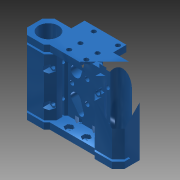
# Autodesk Inventor part: ChimeraXCarriage5
Saved by Autodesk Inventor 2015 SP1 (Build 190203100, 203)
## iProperties
Created: 2015-03-08
Part Number: ChimeraXCarriage5
Material: ABS Plastic
Document SubType Name: Modeling
Designer: Jack
Density: 1.06 g/cm^3
Appearance: Cyan
Author: Jack
Autodesk Inventor part; units mm, degrees
ref_plane "YZ Plane" through (0, 0, 0) normal (1, 0, 0) x (0, 1, 0)
ref_plane "XZ Plane" through (0, 0, 0) normal (0, 1, 0) x (-1, 0, 0)
ref_plane "XY Plane" through (0, 0, 0) normal (0, 0, 1) x (1, 0, 0)
sketch "Sketch2" plane through (0, 0, 0) normal (0, 0, 1) x (1, 0, 0)
  arc A0 (7.6035, 1.5) -> (7.6035, -1.5) centre (0, 0) ccw
  arc A1 (47.3965, -1.5) -> (47.3965, 1.5) centre (55, 0) ccw
  line L0 (-11, -11) -> (-11, 11)
  line L1 (66, 11) -> (66, -11)
  line L2 (66, -11) -> (42.5, -11)
  line L3 (42.5, -11) -> (42.5, -1.5)
  line L4 (42.5, -1.5) -> (47.3965, -1.5)
  line L5 (-11, -11) -> (12.5, -11)
  line L6 (12.5, -11) -> (12.5, -1.5)
  line L7 (7.6035, -1.5) -> (12.5, -1.5)
  line L8 (-11, 11) -> (66, 11)
  line L9 (7.6035, 1.5) -> (12.5, 1.5)
  line L10 (12.5, 1.5) -> (12.5, 3)
  line L11 (12.5, 3) -> (42.5, 3)
  line L12 (42.5, 3) -> (42.5, 1.5)
  line L13 (42.5, 1.5) -> (47.3965, 1.5)
  dimension "d11" = 15.5
  dimension "d12" = 55
  dimension "d13" = 11
  dimension "d15" = 11
  dimension "d17" = 1.5
  dimension "d18" = 12.5
  dimension "d19" = 12.5
  dimension "d20" = 11
  dimension "d29" = 1.5
  dimension "d30" = 8
  constraints: 28 end point, 6 perpendicular, 5 point on circle, 4 horizontal, 3 point on line, 2 centre point, 2 collinear, 2 horizontal alignment, 2 vertical, 1 coincident, 1 equal radius, 1 parallel, 1 vertical alignment
  measures "d11" diameter of A0
  measures "d12" distance of A1.centre point (0, 0)
  measures "d13" distance from line of L5 point (0, 0)
  measures "d15" distance from line of point (0, 0) L0
  measures "d17" distance from line of point (0, 0) L7
  measures "d18" distance from line of point (0, 0) L6
  measures "d19" distance from line of A1.centre L3
  measures "d20" distance from line of point (0, 0) L8
  measures "d29" distance from line of point (0, 0) L9
  measures "d30" distance between parallel lines of L8 L11
extrude "Extrusion1" add sketch "Sketch2" along normal blind 48
chamfer "Chamfer1" distance 5 angle 45 2 edges at (12.5, -11, 24) (42.5, -11, 24)
chamfer "Chamfer2" distance 5 angle 45 4 edges at (-11, -11, 24) (-11, 11, 24) (66, 11, 24) (66, -11, 24)
sketch "Sketch6" plane through (0, 0, 0) normal (0, 0, -1) x (-1, 0, 0)
  line L0 (-61, -11) -> (-66, -6) projected
  line L1 (-61, -11) -> (-47.5, -11) projected
  line L2 (-42.5, -6) -> (-42.5, -1.5) projected
  line L3 (-42.5, -1.5) -> (-47.3965, -1.5) projected
  arc A0 (-47.3965, 1.5) -> (-47.3965, -1.5) centre (-55, 0) ccw projected
  line L4 (-47.3965, 1.5) -> (-42.5, 1.5) projected
  line L5 (-42.5, 1.5) -> (-42.5, 3) projected
  line L6 (-42.5, 3) -> (-12.5, 3) projected
  line L7 (-12.5, 3) -> (-12.5, 1.5) projected
  line L8 (-12.5, 1.5) -> (-7.6035, 1.5) projected
  arc A1 (-7.6035, -1.5) -> (-7.6035, 1.5) centre (0, 0) ccw projected
  line L9 (-7.6035, -1.5) -> (-12.5, -1.5) projected
  line L10 (-12.5, -1.5) -> (-12.5, -6) projected
  line L11 (-7.5, -11) -> (6, -11) projected
  line L12 (11, -6) -> (6, -11) projected
  line L13 (11, -6) -> (11, 6) projected
  line L14 (6, 11) -> (11, 6) projected
  line L15 (6, 11) -> (-61, 11) projected
  line L16 (-66, 6) -> (-61, 11) projected
  line L17 (-66, 6) -> (-66, -6) projected
  line L18 (-47.5, -11) -> (-42.5, -6) projected
  line L19 (-45.2, -8.7) -> (-9.8, -8.7)
  line L20 (-12.5, -6) -> (-7.5, -11) projected
  arc A2 (-47.3965, -1.5) -> (-47.3965, 1.5) centre (-55, 0) ccw
  arc A3 (-7.6035, 1.5) -> (-7.6035, -1.5) centre (0, 0) ccw
  dimension "d37" = 8.7
  constraints: 4 point on circle, 2 centre point, 2 coincident, 2 end point, 2 point on line, 1 horizontal
  measures "d37" distance from line of A0.centre L19
extrude "Extrusion4" add sketch "Sketch6" along normal blind 5 contours L0 L17 L16 L15 L14 L13 L12 L11 L20 L10 L9 A1 L8 L7 L6 L5 L4 A0 L3 L2 L18 L1 | L18 L2 L3 A2 L4 L5 L6 L7 L8 A3 L9 L10 L20 L19
sketch "Sketch7" plane through (0, 0, 48) normal (0, 0, 1) x (1, 0, 0)
  line L0 (66, -6) -> (61, -11) projected
  line L1 (66, -6) -> (66, 6) projected
  line L2 (61, 11) -> (66, 6) projected
  line L3 (61, 11) -> (-6, 11) projected
  line L4 (-11, 6) -> (-6, 11) projected
  line L5 (-11, 6) -> (-11, -6) projected
  line L6 (-6, -11) -> (-11, -6) projected
  line L7 (-6, -11) -> (7.5, -11) projected
  line L8 (12.5, -6) -> (7.5, -11) projected
  line L9 (12.5, -6) -> (12.5, -1.5) projected
  line L10 (12.5, -1.5) -> (7.6035, -1.5) projected
  arc A0 (7.6035, 1.5) -> (7.6035, -1.5) centre (0, 0) ccw projected
  line L11 (7.6035, 1.5) -> (12.5, 1.5) projected
  line L12 (12.5, 1.5) -> (12.5, 3) projected
  line L13 (12.5, 3) -> (42.5, 3) projected
  line L14 (42.5, 3) -> (42.5, 1.5) projected
  line L15 (42.5, 1.5) -> (47.3965, 1.5) projected
  arc A1 (47.3965, -1.5) -> (47.3965, 1.5) centre (55, 0) ccw projected
  line L16 (47.3965, -1.5) -> (42.5, -1.5) projected
  line L17 (42.5, -1.5) -> (42.5, -6) projected
  line L18 (47.5, -11) -> (42.5, -6) projected
  line L19 (47.5, -11) -> (61, -11) projected
  line L20 (42.5, -6) -> (45.2, -8.7) projected
  line L21 (42.5, -6) -> (42.5, -1.5) projected
  line L22 (42.5, -1.5) -> (47.3965, -1.5) projected
  arc A2 (47.3965, 1.5) -> (47.3965, -1.5) centre (55, 0) ccw projected
  line L23 (47.3965, 1.5) -> (42.5, 1.5) projected
  line L24 (42.5, 1.5) -> (42.5, 3) projected
  line L25 (42.5, 3) -> (12.5, 3) projected
  line L26 (12.5, 3) -> (12.5, 1.5) projected
  line L27 (12.5, 1.5) -> (7.6035, 1.5) projected
  arc A3 (7.6035, -1.5) -> (7.6035, 1.5) centre (0, 0) ccw projected
  line L28 (7.6035, -1.5) -> (12.5, -1.5) projected
  line L29 (12.5, -1.5) -> (12.5, -6) projected
  line L30 (9.8, -8.7) -> (12.5, -6) projected
  line L31 (45.2, -8.7) -> (9.8, -8.7) projected
extrude "Extrusion5" add sketch "Sketch7" along normal blind 5 contours L0 L19 L18 L17 L16 A1 L15 L14 L13 L12 L11 A0 L10 L9 L8 L7 L6 L5 L4 L3 L2 L1 | L31 L8 L9 L10 A3 L11 L12 L13 L14 L15 A2 L16 L17 L18
sketch "Sketch8" plane through (-11, -6, -5) normal (-1, 0, 0) x (0, 0, 1)
  line L0 (5, 4.5) -> (53, 4.5) projected
  line L1 (0, -5) -> (58, -5) projected
  line L2 (53, 4.5) -> (53, -5)
  line L3 (58, -5) -> (0, -5) projected
  line L4 (51.5, 4.5) -> (51.5, -5)
  point P0 (5, 6)
  dimension "d42" = 1.5
  constraints: 4 end point, 3 point on line, 2 perpendicular
  measures "d42" distance between parallel lines of L2 L4
extrude "Extrusion6" cut sketch "Sketch8" against normal up to surface (23.5 mm away)
sketch "Sketch9" plane through (-11, -6, -5) normal (-1, 0, 0) x (0, 0, 1)
  line L0 (0, -5) -> (51.5, -5) projected
  line L1 (5, 4.5) -> (51.5, 4.5) projected
  line L2 (6.5, 4.5) -> (6.5, -5)
  line L3 (51.5, -5) -> (0, -5) projected
  line L4 (5, 4.5) -> (5, -5)
  point P0 (5, 6)
  dimension "d45" = 1.5
  constraints: 4 end point, 3 point on line, 2 perpendicular
  measures "d45" distance between parallel lines of L4 L2
extrude "Extrusion7" cut sketch "Sketch9" against normal up to surface (23.5 mm away)
sketch "Sketch10" plane through (66, -6, -5) normal (1, 0, 0) x (0, 0, -1)
  line L0 (-5, 4.5) -> (-53, 4.5) projected
  line L1 (-58, -5) -> (0, -5) projected
  line L2 (-53, 4.5) -> (-53, -5)
  line L3 (-53, -5) -> (-53, -2.7) projected
  line L4 (-5, 4.5) -> (-5, -5)
  line L5 (0, -5) -> (-58, -5) projected
  line L6 (-6.5, 4.5) -> (-51.5, 4.5) projected
  line L7 (-6.5, 4.5) -> (-6.5, -5)
  line L8 (-51.5, -5) -> (-6.5, -5) projected
  line L9 (-51.5, 4.5) -> (-51.5, -5)
  point P0 (-5, 6)
  dimension "d48" = 1.5
  dimension "d49" = 1.5
  constraints: 8 end point, 5 point on line, 2 perpendicular, 1 collinear, 1 vertical
  measures "d48" distance between parallel lines of L2 L9
  measures "d49" distance between parallel lines of L4 L7
extrude "Extrusion8" cut sketch "Sketch10" against normal up to surface (23.5 mm away) contours L4 L1 L7 L0 | L9 L1 L2 L0
chamfer "Chamfer3" distance 1.5 angle 45 2 edges at (12.5, 1.5, 24) (42.5, 1.5, 24)
sketch "Sketch11" plane through (-6, -11, 46.5) normal (0, -1, 0) x (1, 0, 0)
  line L0 (18.5, -45) -> (18.5, 0) projected
  line L1 (48.5, 0) -> (48.5, -45) projected
  line L2 (53.5, -45) -> (53.5, 0) projected
  circle A0 centre (15.5, -10) radius 1.75
  circle A1 centre (15.5, -35) radius 1.75
  circle A2 centre (51, -35) radius 1.75
  circle A3 centre (51, -10) radius 1.75
  line L3 (53.5, 0) -> (48.5, 0) projected
  line L4 (48.5, -45) -> (53.5, -45) projected
  point P0 (6, -46.5)
  dimension "d55" = 3.5
  dimension "d56" = 3
  dimension "d57" = 2.5
  dimension "d58" = 10
  dimension "d59" = 10
  constraints: 4 centre point, 3 equal radius, 2 horizontal alignment, 2 vertical alignment
  measures "d55" diameter of A0
  measures "d56" distance from line of L0 A1.centre
  measures "d57" distance from line of L1 A3.centre
  measures "d58" distance from line of L3 A3.centre
  measures "d59" distance from line of L4 A2.centre
extrude "Extrusion9" cut sketch "Sketch11" against normal up to surface (22 mm away) contours A0 | A1 | A2 | A3
sketch "Sketch12" plane through (-6, 11, -5) normal (0, 1, 0) x (1, 0, 0)
  circle A0 centre (51, -16.5) radius 1.75 projected
  circle A1 centre (51, -41.5) radius 1.75 projected
  circle A2 centre (15.5, -16.5) radius 1.75 projected
  circle A3 centre (15.5, -41.5) radius 1.75 projected
  circle A4 centre (15.5, -16.5) radius 3
  circle A5 centre (15.5, -41.5) radius 3
  circle A6 centre (51, -16.5) radius 3
  circle A7 centre (51, -41.5) radius 3
  point P0 (6, -5)
  dimension "d62" = 6
  constraints: 4 centre point, 4 coincident, 3 equal radius
  measures "d62" diameter of A4
extrude "Extrusion10" cut sketch "Sketch12" against normal blind 3.5
sketch "Sketch13" plane through (-6, -11, 46.5) normal (0, -1, 0) x (1, 0, 0)
  circle A0 centre (15.5, -10) radius 1.75 projected
  circle A1 centre (15.5, -35) radius 1.75 projected
  circle A2 centre (51, -10) radius 1.75 projected
  circle A3 centre (51, -35) radius 1.75 projected
  line L0 (15.5, -6.8246) -> (18.25, -8.4123)
  line L1 (18.25, -8.4123) -> (18.25, -11.5877)
  line L2 (18.25, -11.5877) -> (15.5, -13.1754)
  line L3 (15.5, -13.1754) -> (12.75, -11.5877)
  line L4 (12.75, -11.5877) -> (12.75, -8.4123)
  line L5 (12.75, -8.4123) -> (15.5, -6.8246)
  line L6 (15.5, -31.8246) -> (18.25, -33.4123)
  line L7 (18.25, -33.4123) -> (18.25, -36.5877)
  line L8 (18.25, -36.5877) -> (15.5, -38.1754)
  line L9 (15.5, -38.1754) -> (12.75, -36.5877)
  line L10 (12.75, -36.5877) -> (12.75, -33.4123)
  line L11 (12.75, -33.4123) -> (15.5, -31.8246)
  line L12 (51, -31.8246) -> (53.75, -33.4123)
  line L13 (53.75, -33.4123) -> (53.75, -36.5877)
  line L14 (53.75, -36.5877) -> (51, -38.1754)
  line L15 (51, -38.1754) -> (48.25, -36.5877)
  line L16 (48.25, -36.5877) -> (48.25, -33.4123)
  line L17 (48.25, -33.4123) -> (51, -31.8246)
  line L18 (51, -6.8246) -> (53.75, -8.4123)
  line L19 (53.75, -8.4123) -> (53.75, -11.5877)
  line L20 (53.75, -11.5877) -> (51, -13.1754)
  line L21 (51, -13.1754) -> (48.25, -11.5877)
  line L22 (48.25, -11.5877) -> (48.25, -8.4123)
  line L23 (48.25, -8.4123) -> (51, -6.8246)
  point P0 (6, -46.5)
  dimension "d65" = 5.5
  constraints: 48 end point, 4 coincident, 4 vertical, 3 equal length, 52 other
  measures "d65" distance between parallel lines of L4 L1
extrude "Extrusion11" cut sketch "Sketch13" against normal blind 5 contours A0 | A1 | A2 | A3 | L0 L1 L2 L3 L4 L5 | L6 L7 L8 L9 L10 L11 | L12 L13 L14 L15 L16 L17 | L18 L19 L20 L21 L22 L23
sketch "Sketch14" plane through (47.5, -11, 1.5) normal (0, -1, 0) x (1, 0, 0)
  line L0 (-5, 33.2679) -> (-5, 11.7321) projected
  line L1 (-5, 31.5) -> (-2.5, 31.5)
  line L2 (-2.5, 31.5) -> (-2.5, 13.5)
  line L3 (-2.5, 13.5) -> (-5, 13.5)
  line L4 (-5, 0) -> (0, 0) projected
  line L5 (0, 45) -> (-5, 45) projected
  point P0 (-47.5, -1.5)
  dimension "d68" = 2.5
  dimension "d69" = 13.5
  dimension "d70" = 13.5
  constraints: 6 end point, 2 perpendicular, 2 point on line, 1 horizontal
  measures "d68" distance of L2.end L3.end
  measures "d69" distance between parallel lines of L4 L3
  measures "d70" distance between parallel lines of L5 L1
extrude "Extrusion12" cut sketch "Sketch14" against normal up to surface (9.5 mm away)
chamfer "Chamfer4" distance 1 angle 45 2 edges at (45, -5, 15) (45, -5, 33)
sketch "Sketch15" plane through (12.5, 3, 0) normal (0, -1, 0) x (1, 0, 0)
  line L0 (0, 48) -> (30, 48) projected
  line L1 (0, 0) -> (0, 48) projected
  circle A0 centre (15, 32.5) radius 1.75
  circle A1 centre (15, 15.5) radius 1.75
  circle A2 centre (3, 24) radius 1.75
  point P0 (-12.5, 0)
  dimension "d76" = 3.5
  dimension "d77" = 15
  dimension "d78" = 17
  dimension "d79" = 15.5
  dimension "d116" = 12
  dimension "d117" = 8.5
  constraints: 3 centre point, 2 equal radius, 1 vertical alignment
  measures "d76" diameter of A0
  measures "d77" distance from line of L1 A0.centre
  measures "d78" distance of A1.centre A0.centre
  measures "d79" distance from line of L0 A0.centre
  measures "d116" horizontal distance of A0.centre A2.centre
  measures "d117" vertical distance of A1.centre A2.centre
extrude "Extrusion13" cut sketch "Sketch15" against normal up to next
sketch "Sketch16" plane through (-6, 11, -5) normal (0, 1, 0) x (1, 0, 0)
  circle A0 centre (33.5, -37.5) radius 1.75 projected
  arc A1 (28.327, -36.8365) -> (21.273, -40.3635) centre (24.5, -38) ccw
  arc A2 (21.273, -17.6365) -> (28.327, -21.1635) centre (24.5, -20) ccw
  arc A3 (26.4831, -47.4772) -> (30.8919, -45.2728) centre (28.5, -46) ccw
  arc A4 (30.8919, -12.7272) -> (26.4831, -10.5228) centre (28.5, -12) ccw
  line L0 (30.8919, -45.2728) -> (28.327, -36.8365)
  line L1 (26.4831, -47.4772) -> (21.273, -40.3635)
  line L2 (30.8919, -12.7272) -> (28.327, -21.1635)
  line L3 (26.4831, -10.5228) -> (21.273, -17.6365)
  circle A5 centre (21.5, -29) radius 1.75 projected
  point P0 (6, -5)
  dimension "d82" = 8
  dimension "d86" = 5
  dimension "d87" = 8
  dimension "d88" = 4
  dimension "d89" = 8
  dimension "d119" = 18
  dimension "d120" = 9
  dimension "d121" = 9
  constraints: 8 end point, 8 point on circle, 8 tangent, 4 centre point, 2 equal radius, 2 vertical alignment
  measures "d82" diameter of A1
  measures "d86" diameter of A3
  measures "d87" vertical distance of A2.centre A4.centre
  measures "d88" horizontal distance of A2.centre A4.centre
  measures "d89" vertical distance of A1.centre A3.centre
  measures "d119" distance of A2.centre A1.centre
  measures "d120" vertical distance of A5.centre A1.centre
  measures "d121" horizontal distance of A0.centre A1.centre
extrude "Extrusion14" cut sketch "Sketch16" against normal up to next contours L0 A3 L1 A1 | L3 A4 L2 A2
sketch "Sketch17" plane through (-6, 11, -5) normal (0, 1, 0) x (1, 0, 0)
  circle A0 centre (33.5, -37.5) radius 1.75 projected
  circle A1 centre (33.5, -20.5) radius 1.75 projected
  circle A2 centre (33.5, -37.5) radius 3
  circle A3 centre (33.5, -20.5) radius 3
  circle A4 centre (21.5, -29) radius 1.75 projected
  circle A5 centre (21.5, -29) radius 3
  point P0 (6, -5)
  dimension "d90" = 6
  constraints: 3 centre point, 3 coincident, 2 equal radius
  measures "d90" diameter of A2
extrude "Extrusion15" cut sketch "Sketch17" against normal blind 3.5
sketch "Sketch18" plane through (0, 0, 53) normal (0, 0, 1) x (1, 0, 0)
  circle A0 centre (0, 0) radius 7.75 projected
  circle A1 centre (20.75, -4.45) radius 1.75
  circle A2 centre (34.25, -4.45) radius 1.75
  circle A3 centre (34.25, 4.45) radius 1.75
  circle A4 centre (20.75, 4.45) radius 1.75
  dimension "d93" = 3.5
  dimension "d94" = 13.5
  dimension "d95" = 8.9
  dimension "d96" = 20.75
  dimension "d97" = 4.45
  constraints: 4 centre point, 3 equal radius, 2 horizontal alignment, 2 vertical alignment
  measures "d93" diameter of A1
  measures "d94" distance of A3.centre A4.centre
  measures "d95" distance of A4.centre A1.centre
  measures "d96" horizontal distance of A0.centre A1.centre
  measures "d97" vertical distance of A0.centre A1.centre
extrude "Extrusion16" cut sketch "Sketch18" against normal up to surface (5 mm away) contours A1 | A2 | A3 | A4
sketch "Sketch19" plane through (0, 0, -5) normal (0, 0, -1) x (-1, 0, 0)
  circle A0 centre (-20.75, -4.45) radius 1.75 projected
  circle A1 centre (-20.75, 4.45) radius 1.75 projected
  circle A2 centre (-34.25, 4.45) radius 1.75 projected
  circle A3 centre (-34.25, -4.45) radius 1.75 projected
extrude "Extrusion17" cut sketch "Sketch19" against normal up to surface (5 mm away)
sketch "Sketch20" plane through (20.75, 4.45, 0) normal (0, 0, -1) x (-1, 0, 0)
  line L0 (-0.9798, -1.45) -> (0.9798, -1.45) projected
  arc A0 (0.9798, -1.45) -> (-0.9798, -1.45) centre (0, 0) ccw projected
  line L1 (-14.4798, -1.45) -> (-12.5202, -1.45) projected
  arc A1 (-12.5202, -1.45) -> (-14.4798, -1.45) centre (-13.5, 0) ccw projected
  line L2 (-10.75, -1.5877) -> (-13.5, -3.1754)
  line L3 (-13.5, -3.1754) -> (-16.25, -1.5877)
  line L4 (-16.25, -1.5877) -> (-16.25, 1.5877)
  line L5 (-16.25, 1.5877) -> (-13.5, 3.1754)
  line L6 (-13.5, 3.1754) -> (-10.75, 1.5877)
  line L7 (-10.75, 1.5877) -> (-10.75, -1.5877)
  line L8 (-2.75, -1.5877) -> (-2.75, 1.5877)
  line L9 (-2.75, 1.5877) -> (0, 3.1754)
  line L10 (0, 3.1754) -> (2.75, 1.5877)
  line L11 (2.75, 1.5877) -> (2.75, -1.5877)
  line L12 (2.75, -1.5877) -> (0, -3.1754)
  line L13 (0, -3.1754) -> (-2.75, -1.5877)
  point P0 (20.75, -4.45)
  point P1 (-13.5, 0)
  dimension "d102" = 5.5
  constraints: 24 end point, 2 coincident, 2 vertical, 1 parallel, 26 other
  measures "d102" distance between parallel lines of L3 L6
extrude "Extrusion18" cut sketch "Sketch20" along normal blind 3 and the other way blind 3 contours A0 L0 | A1 L1 | L2 L3 L4 L5 L6 L7 | L8 L9 L10 L11 L12 L13
sketch "Sketch21" plane through (34.25, 4.45, 48) normal (0, 0, 1) x (1, 0, 0)
  line L0 (-14.4798, -1.45) -> (-12.5202, -1.45) projected
  arc A0 (-12.5202, -1.45) -> (-14.4798, -1.45) centre (-13.5, 0) ccw projected
  circle A1 centre (-13.5, 0) radius 1.75 projected
  line L1 (-10.75, 1.5877) -> (-10.75, -1.5877) projected
  line L2 (-13.5, 3.1754) -> (-10.75, 1.5877) projected
  line L3 (-16.25, 1.5877) -> (-13.5, 3.1754) projected
  line L4 (-16.25, -1.5877) -> (-16.25, 1.5877) projected
  line L5 (-13.5, -3.1754) -> (-16.25, -1.5877) projected
  line L6 (-10.75, -1.5877) -> (-13.5, -3.1754) projected
  circle A2 centre (0, 0) radius 1.75 projected
  line L7 (0, -3.1754) -> (-2.75, -1.5877) projected
  line L8 (2.75, -1.5877) -> (0, -3.1754) projected
  line L9 (2.75, 1.5877) -> (2.75, -1.5877) projected
  line L10 (0, 3.1754) -> (2.75, 1.5877) projected
  line L11 (-2.75, 1.5877) -> (0, 3.1754) projected
  line L12 (-2.75, -1.5877) -> (-2.75, 1.5877) projected
  point P0 (-34.25, -4.45)
extrude "Extrusion19" cut sketch "Sketch21" along normal blind 3 and the other way blind 3 contours A0 L0 | L1 L6 L5 L4 L3 L2 | A2 | L7 L12 L11 L10 L9 L8
sketch "Sketch22" plane through (0, 0, 48) normal (0, 0, -1) x (-1, 0, 0)
  circle A0 centre (-20.75, -4.45) radius 1.75 projected
  circle A1 centre (-34.25, -4.45) radius 1.75 projected
  line L0 (-18, 2.8623) -> (-20.75, 1.2746) projected
  line L1 (-20.75, -7.6254) -> (-23.5, -6.0377)
  line L2 (-23.5, -6.0377) -> (-23.5, -2.8623)
  line L3 (-23.5, -2.8623) -> (-20.75, -1.2746)
  line L4 (-20.75, -1.2746) -> (-18, -2.8623)
  line L5 (-18, -2.8623) -> (-18, -6.0377)
  line L6 (-18, -6.0377) -> (-20.75, -7.6254)
  line L7 (-34.25, -7.6254) -> (-37, -6.0377)
  line L8 (-37, -6.0377) -> (-37, -2.8623)
  line L9 (-37, -2.8623) -> (-34.25, -1.2746)
  line L10 (-34.25, -1.2746) -> (-31.5, -2.8623)
  line L11 (-31.5, -2.8623) -> (-31.5, -6.0377)
  line L12 (-31.5, -6.0377) -> (-34.25, -7.6254)
  constraints: 24 end point, 2 coincident, 2 equal length, 2 vertical, 26 other
extrude "Extrusion20" cut sketch "Sketch22" against normal blind 3
sketch "Sketch23" plane through (0, 0, 0) normal (0, 0, 1) x (1, 0, 0)
  circle A0 centre (20.75, -4.45) radius 1.75 projected
  circle A1 centre (34.25, -4.45) radius 1.75 projected
  circle A2 centre (20.75, -4.45) radius 1.75 projected
  line L0 (20.75, -7.6254) -> (23.5, -6.0377) projected
  line L1 (18, -6.0377) -> (20.75, -7.6254) projected
  line L2 (18, -2.8623) -> (18, -6.0377) projected
  line L3 (20.75, -1.2746) -> (18, -2.8623) projected
  line L4 (23.5, -2.8623) -> (20.75, -1.2746) projected
  line L5 (23.5, -6.0377) -> (23.5, -2.8623) projected
  circle A3 centre (34.25, -4.45) radius 1.75 projected
  line L6 (34.25, -7.6254) -> (37, -6.0377) projected
  line L7 (31.5, -6.0377) -> (34.25, -7.6254) projected
  line L8 (31.5, -2.8623) -> (31.5, -6.0377) projected
  line L9 (34.25, -1.2746) -> (31.5, -2.8623) projected
  line L10 (37, -2.8623) -> (34.25, -1.2746) projected
  line L11 (37, -6.0377) -> (37, -2.8623) projected
extrude "Extrusion21" cut sketch "Sketch23" against normal blind 3
sketch "Sketch24" plane through (0, 0, 53) normal (0, 0, 1) x (1, 0, 0)
  line L0 (66, -6) -> (66, 6) projected
  line L1 (61, 11) -> (-6, 11) projected
  line L2 (-6, 11) -> (61, 11) projected
  line L3 (7, 11) -> (7, 21.5)
  line L4 (7, 21.5) -> (40, 21.5)
  line L5 (40, 21.5) -> (40, 11)
  dimension "d122" = 33
  dimension "d123" = 26
  dimension "d124" = 10.5
  constraints: 6 end point, 3 perpendicular, 2 point on line
  measures "d122" distance of L3.end L4.end
  measures "d123" distance between parallel lines of L0 L5
  measures "d124" distance of L3.start L3.end
extrude "Extrusion22" add sketch "Sketch24" against normal blind 5
sketch "Sketch25" plane through (0, 0, 53) normal (0, 0, 1) x (1, 0, 0)
  line L0 (40, 11) -> (40, 21.5) projected
  line L1 (40, 21.5) -> (7, 21.5) projected
  circle A0 centre (37, 17.75) radius 1.75
  circle A1 centre (18, 17.75) radius 1.75
  dimension "d127" = 3.5
  dimension "d128" = 3
  dimension "d129" = 19
  dimension "d130" = 3.75
  constraints: 2 centre point, 1 equal radius, 1 horizontal alignment
  measures "d127" diameter of A0
  measures "d128" distance from line of L0 A0.centre
  measures "d129" distance of A0.centre A1.centre
  measures "d130" distance from line of L1 A1.centre
extrude "Extrusion23" cut sketch "Sketch25" against normal up to next
body "Solid1"
